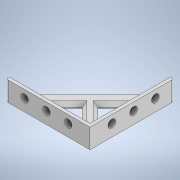
# Autodesk Inventor part: equerre_droite
Saved by Autodesk Inventor 2020 (Build 240168000, 168)
## iProperties
Created: 2020-06-09
Part Number: equerre_droite
Material: Generic
Document SubType Name: Modeling
Designer: Admin
Density: 1 g/cm^3
Appearance: Default
Author: Admin
Autodesk Inventor part; units mm, degrees
ref_plane "YZ Plane" through (0, 0, 0) normal (1, 0, 0) x (0, 1, 0)
ref_plane "XZ Plane" through (0, 0, 0) normal (0, 1, 0) x (-1, 0, 0)
ref_plane "XY Plane" through (0, 0, 0) normal (0, 0, 1) x (1, 0, 0)
sketch "Sketch1" plane through (0, 0, 0) normal (0, 1, 0) x (-1, 0, 0)
  line L0 (0, 0) -> (40, 0)
  line L1 (40, 0) -> (0, -40)
  line L2 (0, -40) -> (0, 0)
  dimension "d0" = 40
  dimension "d1" = 40
  constraints: 6 end point, 1 horizontal, 1 perpendicular
  measures "d0" distance of L0.start L0.end
  measures "d1" distance of L1.end L0.start
extrude "Extrusion1" add sketch "Sketch1" along normal blind 9
sketch "Sketch2" plane through (0, 9, 0) normal (0, 1, 0) x (1, 0, 0)
  line L0 (-37, 3) -> (-3, 3)
  line L1 (-3, 3) -> (-3, 37)
  line L2 (-3, 37) -> (-37, 3)
  line L3 (0, 0) -> (0, 40) projected
  line L4 (-40, 0) -> (0, 0) projected
  line L5 (0, 40) -> (-40, 0) projected
  dimension "d4" = 3
  dimension "d5" = 3
  constraints: 6 end point, 2 point on line, 1 horizontal, 1 perpendicular
  measures "d4" distance between parallel lines of L3 L1
  measures "d5" distance between parallel lines of L4 L0
extrude "Extrusion2" cut sketch "Sketch2" against normal blind 7 contours L2 L1 L0
sketch "Sketch3" plane through (0, 2, 0) normal (0, 1, 0) x (1, 0, 0)
  line L0 (-24.9289, 8) -> (-11.5363, 8)
  line L1 (-11.5363, 8) -> (-18.2326, 14.6963)
  line L2 (-18.2326, 14.6963) -> (-24.9289, 8)
  line L3 (-37, 3) -> (-3, 37) projected
  line L4 (-3, 3) -> (-37, 3) projected
  line L5 (-8, 11.5357) -> (-8, 24.9289)
  line L6 (-8, 24.9289) -> (-14.6966, 18.2323)
  line L7 (-14.6966, 18.2323) -> (-8, 11.5357)
  line L8 (-3, 37) -> (-3, 3) projected
  line L9 (-40, 0) -> (0, 0) projected
  line L10 (0, 0) -> (0, 40) projected
  dimension "d8" = 5
  dimension "d9" = 5
  dimension "d10" = 5
  dimension "d11" = 5
  dimension "d12" = 45
  dimension "d13" = 45
  dimension "d14" = 21.5415
  dimension "d16" = 9.47
  constraints: 12 end point, 2 parallel, 1 horizontal, 1 vertical
  measures "d8" distance between parallel lines of L3 L2
  measures "d9" distance between parallel lines of L0 L4
  measures "d10" distance between parallel lines of L3 L6
  measures "d11" distance between parallel lines of L8 L5
  measures "d12" angle of L1 L9
  measures "d13" angle of L10 L7
  measures "d14" distance from line of L7 L3.end
  measures "d16" distance of L0.end L1.end
extrude "Extrusion3" cut sketch "Sketch3" against normal through all contours L2 L1 L0 | L7 L6 L5
sketch "Sketch4" plane through (0, 0, 0) normal (1, 0, 0) x (0, 0, -1)
  circle A0 centre (10, 5.5) radius 1.75
  circle A1 centre (20, 5.5) radius 1.75
  line L0 (0, 0) -> (40, 0) projected
  circle A2 centre (30, 5.5) radius 1.75
  line L1 (0, 0) -> (0, 9) projected
  line L2 (40, 0) -> (40, 9) projected
  dimension "d19" = 3.5
  dimension "d20" = 3.5
  dimension "d21" = 5.5
  dimension "d22" = 5.5
  dimension "d23" = 3.5
  dimension "d24" = 5.5
  dimension "d25" = 20
  dimension "d26" = 10
  dimension "d27" = 10
  constraints: 3 centre point
  measures "d19" diameter of A0
  measures "d20" diameter of A1
  measures "d21" distance from line of L0 A0.centre
  measures "d22" distance from line of L0 A1.centre
  measures "d23" diameter of A2
  measures "d24" distance from line of L0 A2.centre
  measures "d25" distance from line of L1 A1.centre
  measures "d26" distance from line of L1 A0.centre
  measures "d27" distance from line of L2 A2.centre
sketch "Sketch5" plane through (-40, 0, 0) normal (0, 0, 1) x (1, 0, 0)
  circle A0 centre (10, 5.5) radius 1.75
  circle A1 centre (20, 5.5) radius 1.75
  circle A2 centre (30, 5.5) radius 1.75
  line L0 (0, 0) -> (40, 0) projected
  line L1 (40, 0) -> (40, 9) projected
  line L2 (0, 0) -> (0, 9) projected
  dimension "d30" = 3.5
  dimension "d31" = 3.5
  dimension "d32" = 3.5
  dimension "d33" = 5.5
  dimension "d34" = 5.5
  dimension "d35" = 10
  dimension "d36" = 5.5
  dimension "d37" = 20
  dimension "d38" = 10
  constraints: 3 centre point
  measures "d30" diameter of A0
  measures "d31" diameter of A1
  measures "d32" diameter of A2
  measures "d33" distance from line of L0 A0.centre
  measures "d34" distance from line of L0 A1.centre
  measures "d35" distance from line of L1 A2.centre
  measures "d36" distance from line of L0 A2.centre
  measures "d37" distance from line of L1 A1.centre
  measures "d38" distance from line of L2 A0.centre
extrude "Extrusion6" cut sketch "Sketch4" against normal through all
extrude "Extrusion7" cut sketch "Sketch5" against normal through all
fillet "Fillet1" radius 1 2 edges at (0, 4.5, -40) (-40, 4.5, 0)
chamfer "Chamfer1" distance 1.5 angle 45 8 edges at (-21.5808, 2, -11.3482) (-18.2326, 2, -8) (-14.8845, 2, -11.3482) (-11.3483, 2, -14.884) (-11.3483, 2, -21.5806) (-8, 2, -18.2323) (-20, 9, -3) (-3, 9, -20)
chamfer "Chamfer2" distance 1 angle 45 6 edges at (-31.75, 5.5, -3) (-21.75, 5.5, -3) (-11.75, 5.5, -3) (-3, 5.5, -8.25) (-3, 5.5, -18.25) (-3, 5.5, -28.25)
body "Solid1"
